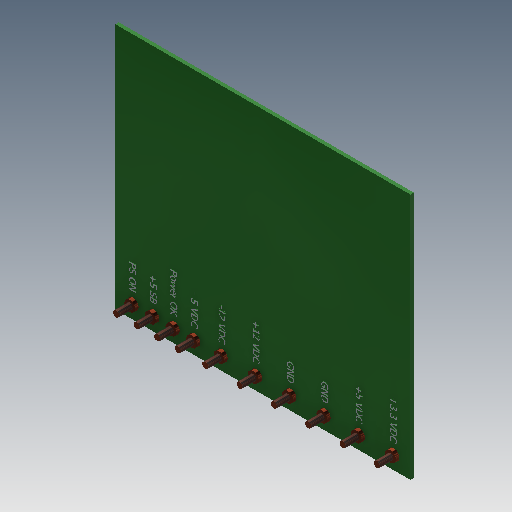
# Autodesk Inventor part: Power Supply PCB
Saved by Autodesk Inventor 2019.1 (Build 231200000, 200)
## iProperties
Created: 2006-09-22
Part Number: Power Supply PCB
Document SubType Name: Modeling
Designer: floress
Density: 1 g/cm^3
Material: Generic
Mass: 25.5294 g
Surface Area: 329.972 cm^2
Volume: 25.5294 cm^3
Appearance: Smooth - Dark Forest Green
Author: floress
Autodesk Inventor part; units mm, degrees
(part 1 of 2)
ref_plane "YZ Plane" through (0, 0, 0) normal (1, 0, 0) x (0, 1, 0)
ref_plane "XZ Plane" through (0, 0, 0) normal (0, 1, 0) x (-1, 0, 0)
ref_plane "XY Plane" through (0, 0, 0) normal (0, 0, 1) x (1, 0, 0)
sketch "Sketch1" plane through (0, 0, 0) normal (0, 0, 1) x (1, 0, 0)
  line L0 (-70.6268, 69.974) -> (65.8982, 69.974)
  line L1 (65.8982, 69.974) -> (65.8982, -44.326)
  line L2 (65.8982, -44.326) -> (-70.6268, -44.326)
  line L3 (-70.6268, -44.326) -> (-70.6268, 69.974)
  circle A0 centre (58.2782, -37.976) radius 2.54
  circle A1 centre (42.4032, -37.976) radius 2.54
  circle A2 centre (26.5282, -37.976) radius 2.54
  circle A3 centre (10.6532, -37.976) radius 2.54
  circle A4 centre (-5.2218, -37.976) radius 2.54
  circle A5 centre (-21.0968, -37.976) radius 2.54
  circle A6 centre (-33.7968, -37.976) radius 2.54
  circle A7 centre (-43.3218, -37.976) radius 2.54
  circle A8 centre (-62.3718, -37.976) radius 2.54
  circle A9 centre (-52.8468, -37.976) radius 2.54
  circle A10 centre (-62.3718, -37.976) radius 1.4224
  circle A11 centre (-52.8468, -37.976) radius 1.4224
  circle A12 centre (-43.3218, -37.976) radius 1.4224
  circle A13 centre (-33.7968, -37.976) radius 1.4224
  circle A14 centre (-21.0968, -37.976) radius 1.4224
  circle A15 centre (-5.2218, -37.976) radius 1.4224
  circle A16 centre (10.6532, -37.976) radius 1.4224
  circle A17 centre (26.5282, -37.976) radius 1.4224
  circle A18 centre (42.4032, -37.976) radius 1.4224
  circle A19 centre (58.2782, -37.976) radius 1.4224
  dimension "d0" = 5.08
  dimension "d1" = 6.35
  dimension "d2" = 7.62
  dimension "d3" = 136.525
  dimension "d4" = 114.3
  dimension "d5" = 15.875
  dimension "d6" = 15.875
  dimension "d7" = 15.875
  dimension "d8" = 15.875
  dimension "d9" = 15.875
  dimension "d10" = 12.7
  dimension "d11" = 9.525
  dimension "d12" = 9.525
  dimension "d13" = 9.525
  dimension "d14" = 2.8448
  constraints: 20 centre point, 18 equal radius, 10 coincident, 9 horizontal alignment, 8 end point, 2 parallel, 1 horizontal, 1 perpendicular
  measures "d0" diameter of A9
  measures "d1" distance from line of L2 A4.centre
  measures "d2" distance from line of L1 A0.centre
  measures "d3" distance of L1.end L2.end
  measures "d4" distance of L0.end L1.end
  measures "d5" distance of A1.centre A0.centre
  measures "d6" distance of A2.centre A1.centre
  measures "d7" distance of A3.centre A2.centre
  measures "d8" distance of A4.centre A3.centre
  measures "d9" distance of A5.centre A4.centre
  measures "d10" distance of A6.centre A5.centre
  measures "d11" distance of A7.centre A6.centre
  measures "d12" distance of A9.centre A7.centre
  measures "d13" distance of A8.centre A9.centre
  measures "d14" diameter of A10
extrude "Extrusion1" add sketch "Sketch1" along normal blind 1.5875 contours L0 L1 L2 L3 | A0 | A1 | A2 | A3 | A4 | A5 | A6 | A7 | A8 | A9 | A10 | A11 | A12 | A13 | A14 | A15 | A16 | A17 | A18 | A19
extrude "Extrusion2" add sketch "Sketch1" along normal blind 3.175 contours A0 | A1 | A2 | A3 | A4 | A5 | A6 | A7 | A8 | A9 | A10 | A11 | A12 | A13 | A14 | A15 | A16 | A17 | A18 | A19
extrude "Extrusion3" add sketch "Sketch1" along normal blind 9.525 contours A10 | A11 | A12 | A13 | A14 | A15 | A16 | A17 | A18 | A19
thread "Thread1" size "4-40 UNC" class "2A" standard "ANSI Unified Screw Threads" full length
thread "Thread2" size "4-40 UNC" class "2A" standard "ANSI Unified Screw Threads" full length
thread "Thread3" size "4-40 UNC" class "2A" standard "ANSI Unified Screw Threads" full length
thread "Thread4" size "4-40 UNC" class "2A" standard "ANSI Unified Screw Threads" full length
thread "Thread5" size "4-40 UNC" class "2A" standard "ANSI Unified Screw Threads" full length
thread "Thread6" size "4-40 UNC" class "2A" standard "ANSI Unified Screw Threads" full length
thread "Thread7" size "4-40 UNC" class "2A" standard "ANSI Unified Screw Threads" full length
thread "Thread8" size "4-40 UNC" class "2A" standard "ANSI Unified Screw Threads" full length
thread "Thread9" size "4-40 UNC" class "2A" standard "ANSI Unified Screw Threads" full length
thread "Thread10" size "4-40 UNC" class "2A" standard "ANSI Unified Screw Threads" full length
sketch "Sketch2" plane through (0, 0, 1.5875) normal (0, 0, 1) x (1, 0, 0)
  circle A0 centre (-52.8468, -37.976) radius 2.54 projected
  circle A1 centre (-62.3718, -37.976) radius 2.54 projected
  circle A2 centre (-43.3218, -37.976) radius 2.54 projected
  circle A3 centre (-33.7968, -37.976) radius 2.54 projected
  circle A4 centre (-21.0968, -37.976) radius 2.54 projected
  circle A5 centre (-5.2218, -37.976) radius 2.54 projected
  circle A6 centre (10.6532, -37.976) radius 2.54 projected
  circle A7 centre (26.5282, -37.976) radius 2.54 projected
  circle A8 centre (42.4032, -37.976) radius 2.54 projected
  circle A9 centre (58.2782, -37.976) radius 2.54 projected
  line L0 (65.8982, 69.974) -> (65.8982, -44.326) projected
  line L1 (59.8664, -14.9782) -> (59.8664, -33.0439) construction
  line L2 (59.8664, -33.0439) -> (56.69, -33.0439) construction
  line L3 (56.69, -33.0439) -> (56.69, -14.9782) construction
  line L4 (56.69, -14.9782) -> (59.8664, -14.9782) construction
  line L5 (43.9914, -14.9782) -> (43.9914, -33.0439) construction
  line L6 (43.9914, -33.0439) -> (40.815, -33.0439) construction
  line L7 (40.815, -33.0439) -> (40.815, -14.9782) construction
  line L8 (40.815, -14.9782) -> (43.9914, -14.9782) construction
  line L9 (28.1164, -14.9782) -> (28.1164, -33.0439) construction
  line L10 (28.1164, -33.0439) -> (24.94, -33.0439) construction
  line L11 (24.94, -33.0439) -> (24.94, -14.9782) construction
  line L12 (24.94, -14.9782) -> (28.1164, -14.9782) construction
  line L13 (9.065, -14.9782) -> (12.2414, -14.9782) construction
  line L14 (12.2414, -14.9782) -> (12.2414, -33.0439) construction
  line L15 (12.2414, -33.0439) -> (9.065, -33.0439) construction
  line L16 (9.065, -33.0439) -> (9.065, -14.9782) construction
  line L17 (-6.81, -14.9782) -> (-3.6336, -14.9782) construction
  line L18 (-3.6336, -14.9782) -> (-3.6336, -33.0439) construction
  line L19 (-3.6336, -33.0439) -> (-6.81, -33.0439) construction
  line L20 (-6.81, -33.0439) -> (-6.81, -14.9782) construction
  line L21 (-60.7836, -14.9782) -> (-60.7836, -33.0439) construction
  line L22 (-60.7836, -33.0439) -> (-63.96, -33.0439) construction
  line L23 (-63.96, -33.0439) -> (-63.96, -14.9782) construction
  line L24 (-63.96, -14.9782) -> (-60.7836, -14.9782) construction
  line L25 (-54.435, -14.9782) -> (-51.2586, -14.9782) construction
  line L26 (-51.2586, -14.9782) -> (-51.2586, -33.0439) construction
  line L27 (-51.2586, -33.0439) -> (-54.435, -33.0439) construction
  line L28 (-54.435, -33.0439) -> (-54.435, -14.9782) construction
  line L29 (-44.91, -14.9782) -> (-41.7336, -14.9782) construction
  line L30 (-41.7336, -14.9782) -> (-41.7336, -33.0439) construction
  line L31 (-41.7336, -33.0439) -> (-44.91, -33.0439) construction
  line L32 (-44.91, -33.0439) -> (-44.91, -14.9782) construction
  line L33 (-35.385, -14.9782) -> (-32.2086, -14.9782) construction
  line L34 (-32.2086, -14.9782) -> (-32.2086, -33.0439) construction
  line L35 (-32.2086, -33.0439) -> (-35.385, -33.0439) construction
  line L36 (-35.385, -33.0439) -> (-35.385, -14.9782) construction
  line L37 (-22.685, -14.9782) -> (-19.5086, -14.9782) construction
  line L38 (-19.5086, -14.9782) -> (-19.5086, -33.0439) construction
  line L39 (-19.5086, -33.0439) -> (-22.685, -33.0439) construction
  line L40 (-22.685, -33.0439) -> (-22.685, -14.9782) construction
  line L41 (57.925, -17.7076) -> (57.925, -16.6751)
  line L42 (57.925, -16.6751) -> (56.8925, -16.6751)
  line L43 (56.8925, -16.6751) -> (56.8925, -16.3342)
  line L44 (56.8925, -16.3342) -> (57.925, -16.3342)
  line L45 (57.925, -16.3342) -> (57.925, -15.3018)
  line L46 (57.925, -15.3018) -> (58.2535, -15.3018)
  line L47 (58.2535, -15.3018) -> (58.2535, -16.3342)
  line L48 (58.2535, -16.3342) -> (59.286, -16.3342)
  line L49 (59.286, -16.3342) -> (59.286, -16.6751)
  line L50 (59.286, -16.6751) -> (58.2535, -16.6751)
  line L51 (58.2535, -16.6751) -> (58.2535, -17.7076)
  line L52 (58.2535, -17.7076) -> (57.925, -17.7076)
  spline S0 degree 2 poles (59.5132, -19.0735) (59.5132, -18.9623) (59.4589, -18.7425) (59.4169, -18.6363) knots 0 0 0 1 2 2 2
  spline S1 degree 2 poles (59.4169, -18.6363) (59.3749, -18.5375) (59.286, -18.3918) (59.2464, -18.335) knots 0 0 0 1 2 2 2
  line L53 (59.2464, -18.335) -> (59.2464, -18.3103)
  line L54 (59.2464, -18.3103) -> (59.6787, -18.3103)
  spline S2 degree 2 poles (59.6787, -18.3103) (59.7503, -18.4436) (59.8664, -18.9006) (59.8664, -19.1056) knots 0 0 0 1 2 2 2
  spline S3 degree 2 poles (59.8664, -19.1056) (59.8664, -19.3131) (59.7824, -19.6218) (59.6935, -19.7478) knots 0 0 0 1 2 2 2
  spline S4 degree 2 poles (59.6935, -19.7478) (59.5972, -19.8812) (59.3181, -20.0195) (59.1304, -20.0195) knots 0 0 0 1 2 2 2
  spline S5 degree 2 poles (59.1304, -20.0195) (58.8784, -20.0195) (58.498, -19.6885) (58.4486, -19.4563) knots 0 0 0 1 2 2 2
  line L55 (58.4486, -19.4563) -> (58.419, -19.4563)
  spline S6 degree 2 poles (58.419, -19.4563) (58.3992, -19.5527) (58.3103, -19.7725) (58.2214, -19.8664) knots 0 0 0 1 2 2 2
  spline S7 degree 2 poles (58.2214, -19.8664) (58.1349, -19.9602) (57.8583, -20.0788) (57.6582, -20.0788) knots 0 0 0 1 2 2 2
  spline S8 degree 2 poles (57.6582, -20.0788) (57.4532, -20.0788) (57.1049, -19.938) (56.9716, -19.8096) knots 0 0 0 1 2 2 2
  spline S9 degree 2 poles (56.9716, -19.8096) (56.8332, -19.6762) (56.69, -19.2983) (56.69, -19.0587) knots 0 0 0 1 2 2 2
  spline S10 degree 2 poles (56.69, -19.0587) (56.69, -18.829) (56.8011, -18.3794) (56.8777, -18.2263) knots 0 0 0 1 2 2 2
  line L56 (56.8777, -18.2263) -> (57.31, -18.2263)
  line L57 (57.31, -18.2263) -> (57.31, -18.2559)
  spline S11 degree 2 poles (57.31, -18.2559) (57.2161, -18.3844) (57.0432, -18.8191) (57.0432, -19.034) knots 0 0 0 1 2 2 2
  spline S12 degree 2 poles (57.0432, -19.034) (57.0432, -19.1599) (57.1222, -19.4119) (57.2136, -19.4959) knots 0 0 0 1 2 2 2
  spline S13 degree 2 poles (57.2136, -19.4959) (57.305, -19.5774) (57.5224, -19.6638) (57.6879, -19.6638) knots 0 0 0 1 2 2 2
  spline S14 degree 2 poles (57.6879, -19.6638) (57.8534, -19.6638) (58.0682, -19.5675) (58.13, -19.481) knots 0 0 0 1 2 2 2
  spline S15 degree 2 poles (58.13, -19.481) (58.1917, -19.3946) (58.2387, -19.1599) (58.2387, -19.0216) knots 0 0 0 1 2 2 2
  line L58 (58.2387, -19.0216) -> (58.2387, -18.8487)
  line L59 (58.2387, -18.8487) -> (58.5771, -18.8487)
  line L60 (58.5771, -18.8487) -> (58.5771, -18.9846)
  spline S16 degree 2 poles (58.5771, -18.9846) (58.5771, -19.2587) (58.8389, -19.6045) (59.0884, -19.6045) knots 0 0 0 1 2 2 2
  spline S17 degree 2 poles (59.0884, -19.6045) (59.2045, -19.6045) (59.3699, -19.5156) (59.4193, -19.444) knots 0 0 0 1 2 2 2
  spline S18 degree 2 poles (59.4193, -19.444) (59.4712, -19.3674) (59.5132, -19.1797) (59.5132, -19.0735) knots 0 0 0 1 2 2 2
  line L61 (56.7542, -21.1928) -> (56.7542, -20.7037)
  line L62 (56.7542, -20.7037) -> (57.3371, -20.7037)
  line L63 (57.3371, -20.7037) -> (57.3371, -21.1928)
  line L64 (57.3371, -21.1928) -> (56.7542, -21.1928)
  spline S19 degree 2 poles (59.5132, -22.6303) (59.5132, -22.5192) (59.4589, -22.2993) (59.4169, -22.1931) knots 0 0 0 1 2 2 2
  spline S20 degree 2 poles (59.4169, -22.1931) (59.3749, -22.0943) (59.286, -21.9486) (59.2464, -21.8918) knots 0 0 0 1 2 2 2
  line L65 (59.2464, -21.8918) -> (59.2464, -21.8671)
  line L66 (59.2464, -21.8671) -> (59.6787, -21.8671)
  spline S21 degree 2 poles (59.6787, -21.8671) (59.7503, -22.0005) (59.8664, -22.4574) (59.8664, -22.6624) knots 0 0 0 1 2 2 2
  spline S22 degree 2 poles (59.8664, -22.6624) (59.8664, -22.8699) (59.7824, -23.1787) (59.6935, -23.3046) knots 0 0 0 1 2 2 2
  spline S23 degree 2 poles (59.6935, -23.3046) (59.5972, -23.438) (59.3181, -23.5763) (59.1304, -23.5763) knots 0 0 0 1 2 2 2
  spline S24 degree 2 poles (59.1304, -23.5763) (58.8784, -23.5763) (58.498, -23.2453) (58.4486, -23.0132) knots 0 0 0 1 2 2 2
  line L67 (58.4486, -23.0132) -> (58.419, -23.0132)
  spline S25 degree 2 poles (58.419, -23.0132) (58.3992, -23.1095) (58.3103, -23.3293) (58.2214, -23.4232) knots 0 0 0 1 2 2 2
  spline S26 degree 2 poles (58.2214, -23.4232) (58.1349, -23.5171) (57.8583, -23.6356) (57.6582, -23.6356) knots 0 0 0 1 2 2 2
  spline S27 degree 2 poles (57.6582, -23.6356) (57.4532, -23.6356) (57.1049, -23.4948) (56.9716, -23.3664) knots 0 0 0 1 2 2 2
  spline S28 degree 2 poles (56.9716, -23.3664) (56.8332, -23.233) (56.69, -22.8551) (56.69, -22.6155) knots 0 0 0 1 2 2 2
  spline S29 degree 2 poles (56.69, -22.6155) (56.69, -22.3858) (56.8011, -21.9362) (56.8777, -21.7831) knots 0 0 0 1 2 2 2
  line L68 (56.8777, -21.7831) -> (57.31, -21.7831)
  line L69 (57.31, -21.7831) -> (57.31, -21.8127)
  spline S30 degree 2 poles (57.31, -21.8127) (57.2161, -21.9412) (57.0432, -22.3759) (57.0432, -22.5908) knots 0 0 0 1 2 2 2
  spline S31 degree 2 poles (57.0432, -22.5908) (57.0432, -22.7168) (57.1222, -22.9687) (57.2136, -23.0527) knots 0 0 0 1 2 2 2
  spline S32 degree 2 poles (57.2136, -23.0527) (57.305, -23.1342) (57.5224, -23.2206) (57.6879, -23.2206) knots 0 0 0 1 2 2 2
  spline S33 degree 2 poles (57.6879, -23.2206) (57.8534, -23.2206) (58.0682, -23.1243) (58.13, -23.0379) knots 0 0 0 1 2 2 2
  spline S34 degree 2 poles (58.13, -23.0379) (58.1917, -22.9514) (58.2387, -22.7168) (58.2387, -22.5784) knots 0 0 0 1 2 2 2
  line L70 (58.2387, -22.5784) -> (58.2387, -22.4055)
  line L71 (58.2387, -22.4055) -> (58.5771, -22.4055)
  line L72 (58.5771, -22.4055) -> (58.5771, -22.5414)
  spline S35 degree 2 poles (58.5771, -22.5414) (58.5771, -22.8156) (58.8389, -23.1614) (59.0884, -23.1614) knots 0 0 0 1 2 2 2
  spline S36 degree 2 poles (59.0884, -23.1614) (59.2045, -23.1614) (59.3699, -23.0724) (59.4193, -23.0008) knots 0 0 0 1 2 2 2
  spline S37 degree 2 poles (59.4193, -23.0008) (59.4712, -22.9242) (59.5132, -22.7365) (59.5132, -22.6303) knots 0 0 0 1 2 2 2
  line L73 (59.8022, -27.7013) -> (56.7542, -26.6515)
  line L74 (56.7542, -26.6515) -> (56.7542, -26.2143)
  line L75 (56.7542, -26.2143) -> (59.8022, -25.1646)
  line L76 (59.8022, -25.1646) -> (59.8022, -25.5993)
  line L77 (59.8022, -25.5993) -> (57.2704, -26.444)
  line L78 (57.2704, -26.444) -> (59.8022, -27.2888)
  line L79 (59.8022, -27.2888) -> (59.8022, -27.7013)
  spline S38 degree 2 poles (58.2757, -30.396) (57.8583, -30.396) (57.1865, -30.0577) (56.9987, -29.7736) knots 0 0 0 1 2 2 2
  spline S39 degree 2 poles (56.9987, -29.7736) (56.853, -29.5414) (56.7542, -29.0647) (56.7542, -28.6942) knots 0 0 0 1 2 2 2
  line L80 (56.7542, -28.6942) -> (56.7542, -27.9927)
  line L81 (56.7542, -27.9927) -> (59.8022, -27.9927)
  line L82 (59.8022, -27.9927) -> (59.8022, -28.6868)
  spline S40 degree 2 poles (59.8022, -28.6868) (59.8022, -29.1166) (59.6738, -29.6056) (59.5601, -29.7785) knots 0 0 0 1 2 2 2
  spline S41 degree 2 poles (59.5601, -29.7785) (59.365, -30.0725) (58.7203, -30.396) (58.2757, -30.396) knots 0 0 0 1 2 2 2
  spline S42 degree 2 poles (58.2807, -29.9737) (58.6314, -29.9737) (59.1279, -29.7415) (59.2687, -29.5118) knots 0 0 0 1 2 2 2
  spline S43 degree 2 poles (59.2687, -29.5118) (59.365, -29.3488) (59.4515, -28.9807) (59.4515, -28.7066) knots 0 0 0 1 2 2 2
  line L83 (59.4515, -28.7066) -> (59.4515, -28.3978)
  line L84 (59.4515, -28.3978) -> (57.1049, -28.3978)
  line L85 (57.1049, -28.3978) -> (57.1049, -28.7066)
  spline S44 degree 2 poles (57.1049, -28.7066) (57.1049, -28.9758) (57.1914, -29.3833) (57.3075, -29.5488) knots 0 0 0 1 2 2 2
  spline S45 degree 2 poles (57.3075, -29.5488) (57.4507, -29.7613) (57.925, -29.9737) (58.2807, -29.9737) knots 0 0 0 1 2 2 2
  spline S46 degree 2 poles (56.6999, -32.0263) (56.6999, -31.7299) (56.8999, -31.2284) (57.1, -31.0457) knots 0 0 0 1 2 2 2
  spline S47 degree 2 poles (57.1, -31.0457) (57.2976, -30.8629) (57.8904, -30.6628) (58.2757, -30.6628) knots 0 0 0 1 2 2 2
  spline S48 degree 2 poles (58.2757, -30.6628) (58.6586, -30.6628) (59.2267, -30.8579) (59.4366, -31.0432) knots 0 0 0 1 2 2 2
  spline S49 degree 2 poles (59.4366, -31.0432) (59.6416, -31.226) (59.8565, -31.7249) (59.8565, -32.0337) knots 0 0 0 1 2 2 2
  spline S50 degree 2 poles (59.8565, -32.0337) (59.8565, -32.1868) (59.8121, -32.456) (59.7775, -32.5697) knots 0 0 0 1 2 2 2
  spline S51 degree 2 poles (59.7775, -32.5697) (59.7454, -32.6685) (59.654, -32.8735) (59.5997, -32.9747) knots 0 0 0 1 2 2 2
  line L86 (59.5997, -32.9747) -> (59.1106, -32.9747)
  line L87 (59.1106, -32.9747) -> (59.1106, -32.9426)
  spline S52 degree 2 poles (59.1106, -32.9426) (59.16, -32.8883) (59.2983, -32.7203) (59.365, -32.5993) knots 0 0 0 1 2 2 2
  spline S53 degree 2 poles (59.365, -32.5993) (59.4292, -32.4832) (59.5107, -32.209) (59.5107, -32.0312) knots 0 0 0 1 2 2 2
  spline S54 degree 2 poles (59.5107, -32.0312) (59.5107, -31.8361) (59.3502, -31.4878) (59.197, -31.3569) knots 0 0 0 1 2 2 2
  spline S55 degree 2 poles (59.197, -31.3569) (59.0414, -31.2284) (58.5697, -31.0852) (58.2757, -31.0852) knots 0 0 0 1 2 2 2
  spline S56 degree 2 poles (58.2757, -31.0852) (57.962, -31.0852) (57.51, -31.2359) (57.3544, -31.3668) knots 0 0 0 1 2 2 2
  spline S57 degree 2 poles (57.3544, -31.3668) (57.2037, -31.4952) (57.0506, -31.8385) (57.0506, -32.0312) knots 0 0 0 1 2 2 2
  spline S58 degree 2 poles (57.0506, -32.0312) (57.0506, -32.2066) (57.1371, -32.5054) (57.2013, -32.6215) knots 0 0 0 1 2 2 2
  spline S59 degree 2 poles (57.2013, -32.6215) (57.2655, -32.7327) (57.3989, -32.8982) (57.4458, -32.9451) knots 0 0 0 1 2 2 2
  line L88 (57.4458, -32.9451) -> (57.4458, -32.9747)
  line L89 (57.4458, -32.9747) -> (56.9617, -32.9747)
  spline S60 degree 2 poles (56.9617, -32.9747) (56.9147, -32.8735) (56.8283, -32.6956) (56.7888, -32.5697) knots 0 0 0 1 2 2 2
  spline S61 degree 2 poles (56.7888, -32.5697) (56.7443, -32.4363) (56.6999, -32.209) (56.6999, -32.0263) knots 0 0 0 1 2 2 2
  line L90 (42.0599, -21.2644) -> (42.0599, -20.2319)
  line L91 (42.0599, -20.2319) -> (41.0274, -20.2319)
  line L92 (41.0274, -20.2319) -> (41.0274, -19.8911)
  line L93 (41.0274, -19.8911) -> (42.0599, -19.8911)
  line L94 (42.0599, -19.8911) -> (42.0599, -18.8586)
  line L95 (42.0599, -18.8586) -> (42.3884, -18.8586)
  line L96 (42.3884, -18.8586) -> (42.3884, -19.8911)
  line L97 (42.3884, -19.8911) -> (43.4208, -19.8911)
  line L98 (43.4208, -19.8911) -> (43.4208, -20.2319)
  line L99 (43.4208, -20.2319) -> (42.3884, -20.2319)
  line L100 (42.3884, -20.2319) -> (42.3884, -21.2644)
  line L101 (42.3884, -21.2644) -> (42.0599, -21.2644)
  spline S62 degree 2 poles (41.8573, -23.6554) (41.6375, -23.6554) (41.2621, -23.5146) (41.1237, -23.3861) knots 0 0 0 1 2 2 2
  spline S63 degree 2 poles (41.1237, -23.3861) (40.9854, -23.2577) (40.8249, -22.8748) (40.8249, -22.6377) knots 0 0 0 1 2 2 2
  spline S64 degree 2 poles (40.8249, -22.6377) (40.8249, -22.4204) (40.9212, -21.9955) (40.9978, -21.8399) knots 0 0 0 1 2 2 2
  line L102 (40.9978, -21.8399) -> (41.43, -21.8399)
  line L103 (41.43, -21.8399) -> (41.43, -21.8695)
  spline S65 degree 2 poles (41.43, -21.8695) (41.3954, -21.9165) (41.3065, -22.0919) (41.267, -22.1981) knots 0 0 0 1 2 2 2
  spline S66 degree 2 poles (41.267, -22.1981) (41.225, -22.3191) (41.1781, -22.5192) (41.1781, -22.6451) knots 0 0 0 1 2 2 2
  spline S67 degree 2 poles (41.1781, -22.6451) (41.1781, -22.7686) (41.267, -23.0008) (41.3633, -23.0848) knots 0 0 0 1 2 2 2
  spline S68 degree 2 poles (41.3633, -23.0848) (41.4547, -23.1614) (41.6968, -23.2404) (41.8598, -23.2404) knots 0 0 0 1 2 2 2
  spline S69 degree 2 poles (41.8598, -23.2404) (42.0228, -23.2404) (42.2303, -23.1515) (42.2995, -23.0675) knots 0 0 0 1 2 2 2
  spline S70 degree 2 poles (42.2995, -23.0675) (42.376, -22.9811) (42.4402, -22.7242) (42.4402, -22.5686) knots 0 0 0 1 2 2 2
  spline S71 degree 2 poles (42.4402, -22.5686) (42.4402, -22.4006) (42.3884, -22.0672) (42.3661, -21.9659) knots 0 0 0 1 2 2 2
  line L104 (42.3661, -21.9659) -> (43.9371, -21.9659)
  line L105 (43.9371, -21.9659) -> (43.9371, -23.6381)
  line L106 (43.9371, -23.6381) -> (43.5789, -23.6381)
  line L107 (43.5789, -23.6381) -> (43.5789, -22.3586)
  line L108 (43.5789, -22.3586) -> (42.7663, -22.3586)
  spline S72 degree 2 poles (42.7663, -22.3586) (42.7762, -22.4327) (42.7836, -22.576) (42.7836, -22.6353) knots 0 0 0 1 2 2 2
  spline S73 degree 2 poles (42.7836, -22.6353) (42.7836, -22.8699) (42.707, -23.1935) (42.5934, -23.3417) knots 0 0 0 1 2 2 2
  spline S74 degree 2 poles (42.5934, -23.3417) (42.4798, -23.4924) (42.134, -23.6554) (41.8573, -23.6554) knots 0 0 0 1 2 2 2
  line L109 (43.9371, -27.7013) -> (40.8891, -26.6515)
  line L110 (40.8891, -26.6515) -> (40.8891, -26.2143)
  line L111 (40.8891, -26.2143) -> (43.9371, -25.1646)
  line L112 (43.9371, -25.1646) -> (43.9371, -25.5993)
  line L113 (43.9371, -25.5993) -> (41.4053, -26.444)
  line L114 (41.4053, -26.444) -> (43.9371, -27.2888)
  line L115 (43.9371, -27.2888) -> (43.9371, -27.7013)
  spline S75 degree 2 poles (42.4106, -30.396) (41.9932, -30.396) (41.3213, -30.0577) (41.1336, -29.7736) knots 0 0 0 1 2 2 2
  spline S76 degree 2 poles (41.1336, -29.7736) (40.9879, -29.5414) (40.8891, -29.0647) (40.8891, -28.6942) knots 0 0 0 1 2 2 2
  line L116 (40.8891, -28.6942) -> (40.8891, -27.9927)
  line L117 (40.8891, -27.9927) -> (43.9371, -27.9927)
  line L118 (43.9371, -27.9927) -> (43.9371, -28.6868)
  spline S77 degree 2 poles (43.9371, -28.6868) (43.9371, -29.1166) (43.8086, -29.6056) (43.695, -29.7785) knots 0 0 0 1 2 2 2
  spline S78 degree 2 poles (43.695, -29.7785) (43.4999, -30.0725) (42.8552, -30.396) (42.4106, -30.396) knots 0 0 0 1 2 2 2
  spline S79 degree 2 poles (42.4155, -29.9737) (42.7663, -29.9737) (43.2628, -29.7415) (43.4036, -29.5118) knots 0 0 0 1 2 2 2
  spline S80 degree 2 poles (43.4036, -29.5118) (43.4999, -29.3488) (43.5863, -28.9807) (43.5863, -28.7066) knots 0 0 0 1 2 2 2
  line L119 (43.5863, -28.7066) -> (43.5863, -28.3978)
  line L120 (43.5863, -28.3978) -> (41.2398, -28.3978)
  line L121 (41.2398, -28.3978) -> (41.2398, -28.7066)
  spline S81 degree 2 poles (41.2398, -28.7066) (41.2398, -28.9758) (41.3263, -29.3833) (41.4424, -29.5488) knots 0 0 0 1 2 2 2
  spline S82 degree 2 poles (41.4424, -29.5488) (41.5856, -29.7613) (42.0599, -29.9737) (42.4155, -29.9737) knots 0 0 0 1 2 2 2
  spline S83 degree 2 poles (40.8347, -32.0263) (40.8347, -31.7299) (41.0348, -31.2284) (41.2349, -31.0457) knots 0 0 0 1 2 2 2
  spline S84 degree 2 poles (41.2349, -31.0457) (41.4325, -30.8629) (42.0253, -30.6628) (42.4106, -30.6628) knots 0 0 0 1 2 2 2
  spline S85 degree 2 poles (42.4106, -30.6628) (42.7935, -30.6628) (43.3616, -30.8579) (43.5715, -31.0432) knots 0 0 0 1 2 2 2
  spline S86 degree 2 poles (43.5715, -31.0432) (43.7765, -31.226) (43.9914, -31.7249) (43.9914, -32.0337) knots 0 0 0 1 2 2 2
  spline S87 degree 2 poles (43.9914, -32.0337) (43.9914, -32.1868) (43.947, -32.456) (43.9124, -32.5697) knots 0 0 0 1 2 2 2
  spline S88 degree 2 poles (43.9124, -32.5697) (43.8803, -32.6685) (43.7889, -32.8735) (43.7345, -32.9747) knots 0 0 0 1 2 2 2
  line L122 (43.7345, -32.9747) -> (43.2455, -32.9747)
  line L123 (43.2455, -32.9747) -> (43.2455, -32.9426)
  spline S89 degree 2 poles (43.2455, -32.9426) (43.2949, -32.8883) (43.4332, -32.7203) (43.4999, -32.5993) knots 0 0 0 1 2 2 2
  spline S90 degree 2 poles (43.4999, -32.5993) (43.5641, -32.4832) (43.6456, -32.209) (43.6456, -32.0312) knots 0 0 0 1 2 2 2
  spline S91 degree 2 poles (43.6456, -32.0312) (43.6456, -31.8361) (43.4851, -31.4878) (43.3319, -31.3569) knots 0 0 0 1 2 2 2
  spline S92 degree 2 poles (43.3319, -31.3569) (43.1763, -31.2284) (42.7045, -31.0852) (42.4106, -31.0852) knots 0 0 0 1 2 2 2
  spline S93 degree 2 poles (42.4106, -31.0852) (42.0969, -31.0852) (41.6449, -31.2359) (41.4893, -31.3668) knots 0 0 0 1 2 2 2
  spline S94 degree 2 poles (41.4893, -31.3668) (41.3386, -31.4952) (41.1855, -31.8385) (41.1855, -32.0312) knots 0 0 0 1 2 2 2
  spline S95 degree 2 poles (41.1855, -32.0312) (41.1855, -32.2066) (41.2719, -32.5054) (41.3362, -32.6215) knots 0 0 0 1 2 2 2
  spline S96 degree 2 poles (41.3362, -32.6215) (41.4004, -32.7327) (41.5338, -32.8982) (41.5807, -32.9451) knots 0 0 0 1 2 2 2
  line L124 (41.5807, -32.9451) -> (41.5807, -32.9747)
  line L125 (41.5807, -32.9747) -> (41.0966, -32.9747)
  spline S97 degree 2 poles (41.0966, -32.9747) (41.0496, -32.8735) (40.9632, -32.6956) (40.9237, -32.5697) knots 0 0 0 1 2 2 2
  spline S98 degree 2 poles (40.9237, -32.5697) (40.8792, -32.4363) (40.8347, -32.209) (40.8347, -32.0263) knots 0 0 0 1 2 2 2
  spline S99 degree 2 poles (24.9548, -26.1896) (24.9548, -25.866) (25.1524, -25.33) (25.3525, -25.1374) knots 0 0 0 1 2 2 2
  spline S100 degree 2 poles (25.3525, -25.1374) (25.555, -24.9447) (26.1528, -24.7397) (26.5405, -24.7397) knots 0 0 0 1 2 2 2
  spline S101 degree 2 poles (26.5405, -24.7397) (26.9086, -24.7397) (27.4915, -24.9472) (27.699, -25.1399) knots 0 0 0 1 2 2 2
  spline S102 degree 2 poles (27.699, -25.1399) (27.8991, -25.3251) (28.1164, -25.8685) (28.1164, -26.1921) knots 0 0 0 1 2 2 2
  spline S103 degree 2 poles (28.1164, -26.1921) (28.1164, -26.3477) (28.072, -26.6293) (28.0324, -26.7577) knots 0 0 0 1 2 2 2
  spline S104 degree 2 poles (28.0324, -26.7577) (28.0028, -26.8615) (27.8941, -27.1134) (27.8546, -27.19) knots 0 0 0 1 2 2 2
  line L126 (27.8546, -27.19) -> (27.3655, -27.19)
  line L127 (27.3655, -27.19) -> (27.3655, -27.1554)
  spline S105 degree 2 poles (27.3655, -27.1554) (27.4322, -27.0788) (27.5533, -26.9183) (27.6224, -26.7701) knots 0 0 0 1 2 2 2
  spline S106 degree 2 poles (27.6224, -26.7701) (27.6842, -26.6466) (27.7657, -26.3279) (27.7657, -26.1451) knots 0 0 0 1 2 2 2
  spline S107 degree 2 poles (27.7657, -26.1451) (27.7657, -25.7055) (27.1037, -25.1621) (26.5529, -25.1621) knots 0 0 0 1 2 2 2
  spline S108 degree 2 poles (26.5529, -25.1621) (26.2466, -25.1621) (25.7872, -25.3053) (25.6291, -25.4412) knots 0 0 0 1 2 2 2
  spline S109 degree 2 poles (25.6291, -25.4412) (25.471, -25.5721) (25.3055, -25.9426) (25.3055, -26.1748) knots 0 0 0 1 2 2 2
  spline S110 degree 2 poles (25.3055, -26.1748) (25.3055, -26.3452) (25.3549, -26.6861) (25.4043, -26.8022) knots 0 0 0 1 2 2 2
  line L128 (25.4043, -26.8022) -> (26.1923, -26.8022)
  line L129 (26.1923, -26.8022) -> (26.1923, -26.0957)
  line L130 (26.1923, -26.0957) -> (26.548, -26.0957)
  line L131 (26.548, -26.0957) -> (26.548, -27.2023)
  line L132 (26.548, -27.2023) -> (25.2166, -27.2023)
  spline S111 degree 2 poles (25.2166, -27.2023) (25.182, -27.1257) (25.0758, -26.8639) (25.0437, -26.7528) knots 0 0 0 1 2 2 2
  spline S112 degree 2 poles (25.0437, -26.7528) (24.9993, -26.6021) (24.9548, -26.36) (24.9548, -26.1896) knots 0 0 0 1 2 2 2
  line L133 (25.0141, -29.8922) -> (25.0141, -29.4377)
  line L134 (25.0141, -29.4377) -> (27.6422, -28.0891)
  line L135 (27.6422, -28.0891) -> (25.0141, -28.0891)
  line L136 (25.0141, -28.0891) -> (25.0141, -27.7111)
  line L137 (25.0141, -27.7111) -> (28.0621, -27.7111)
  line L138 (28.0621, -27.7111) -> (28.0621, -28.2867)
  line L139 (28.0621, -28.2867) -> (25.6489, -29.5143)
  line L140 (25.6489, -29.5143) -> (28.0621, -29.5143)
  line L141 (28.0621, -29.5143) -> (28.0621, -29.8922)
  line L142 (28.0621, -29.8922) -> (25.0141, -29.8922)
  spline S113 degree 2 poles (26.5356, -32.913) (26.1182, -32.913) (25.4463, -32.5746) (25.2586, -32.2905) knots 0 0 0 1 2 2 2
  spline S114 degree 2 poles (25.2586, -32.2905) (25.1129, -32.0584) (25.0141, -31.5817) (25.0141, -31.2112) knots 0 0 0 1 2 2 2
  line L143 (25.0141, -31.2112) -> (25.0141, -30.5097)
  line L144 (25.0141, -30.5097) -> (28.0621, -30.5097)
  line L145 (28.0621, -30.5097) -> (28.0621, -31.2037)
  spline S115 degree 2 poles (28.0621, -31.2037) (28.0621, -31.6335) (27.9336, -32.1226) (27.82, -32.2955) knots 0 0 0 1 2 2 2
  spline S116 degree 2 poles (27.82, -32.2955) (27.6249, -32.5894) (26.9802, -32.913) (26.5356, -32.913) knots 0 0 0 1 2 2 2
  spline S117 degree 2 poles (26.5405, -32.4906) (26.8913, -32.4906) (27.3878, -32.2584) (27.5286, -32.0287) knots 0 0 0 1 2 2 2
  spline S118 degree 2 poles (27.5286, -32.0287) (27.6249, -31.8657) (27.7113, -31.4977) (27.7113, -31.2235) knots 0 0 0 1 2 2 2
  line L146 (27.7113, -31.2235) -> (27.7113, -30.9147)
  line L147 (27.7113, -30.9147) -> (25.3648, -30.9147)
  line L148 (25.3648, -30.9147) -> (25.3648, -31.2235)
  spline S119 degree 2 poles (25.3648, -31.2235) (25.3648, -31.4927) (25.4513, -31.9003) (25.5674, -32.0658) knots 0 0 0 1 2 2 2
  spline S120 degree 2 poles (25.5674, -32.0658) (25.7106, -32.2782) (26.1849, -32.4906) (26.5405, -32.4906) knots 0 0 0 1 2 2 2
  spline S121 degree 2 poles (9.0798, -26.1896) (9.0798, -25.866) (9.2774, -25.33) (9.4775, -25.1374) knots 0 0 0 1 2 2 2
  spline S122 degree 2 poles (9.4775, -25.1374) (9.68, -24.9447) (10.2778, -24.7397) (10.6655, -24.7397) knots 0 0 0 1 2 2 2
  spline S123 degree 2 poles (10.6655, -24.7397) (11.0336, -24.7397) (11.6165, -24.9472) (11.824, -25.1399) knots 0 0 0 1 2 2 2
  spline S124 degree 2 poles (11.824, -25.1399) (12.0241, -25.3251) (12.2414, -25.8685) (12.2414, -26.1921) knots 0 0 0 1 2 2 2
  spline S125 degree 2 poles (12.2414, -26.1921) (12.2414, -26.3477) (12.197, -26.6293) (12.1574, -26.7577) knots 0 0 0 1 2 2 2
  spline S126 degree 2 poles (12.1574, -26.7577) (12.1278, -26.8615) (12.0191, -27.1134) (11.9796, -27.19) knots 0 0 0 1 2 2 2
  line L149 (11.9796, -27.19) -> (11.4905, -27.19)
  line L150 (11.4905, -27.19) -> (11.4905, -27.1554)
  spline S127 degree 2 poles (11.4905, -27.1554) (11.5572, -27.0788) (11.6783, -26.9183) (11.7474, -26.7701) knots 0 0 0 1 2 2 2
  spline S128 degree 2 poles (11.7474, -26.7701) (11.8092, -26.6466) (11.8907, -26.3279) (11.8907, -26.1451) knots 0 0 0 1 2 2 2
  spline S129 degree 2 poles (11.8907, -26.1451) (11.8907, -25.7055) (11.2287, -25.1621) (10.6779, -25.1621) knots 0 0 0 1 2 2 2
  spline S130 degree 2 poles (10.6779, -25.1621) (10.3716, -25.1621) (9.9122, -25.3053) (9.7541, -25.4412) knots 0 0 0 1 2 2 2
  spline S131 degree 2 poles (9.7541, -25.4412) (9.596, -25.5721) (9.4305, -25.9426) (9.4305, -26.1748) knots 0 0 0 1 2 2 2
  spline S132 degree 2 poles (9.4305, -26.1748) (9.4305, -26.3452) (9.4799, -26.6861) (9.5293, -26.8022) knots 0 0 0 1 2 2 2
  line L151 (9.5293, -26.8022) -> (10.3173, -26.8022)
  line L152 (10.3173, -26.8022) -> (10.3173, -26.0957)
  line L153 (10.3173, -26.0957) -> (10.673, -26.0957)
  line L154 (10.673, -26.0957) -> (10.673, -27.2023)
  line L155 (10.673, -27.2023) -> (9.3416, -27.2023)
  spline S133 degree 2 poles (9.3416, -27.2023) (9.307, -27.1257) (9.2008, -26.8639) (9.1687, -26.7528) knots 0 0 0 1 2 2 2
  spline S134 degree 2 poles (9.1687, -26.7528) (9.1243, -26.6021) (9.0798, -26.36) (9.0798, -26.1896) knots 0 0 0 1 2 2 2
  line L156 (9.1391, -29.8922) -> (9.1391, -29.4377)
  line L157 (9.1391, -29.4377) -> (11.7672, -28.0891)
  line L158 (11.7672, -28.0891) -> (9.1391, -28.0891)
  line L159 (9.1391, -28.0891) -> (9.1391, -27.7111)
  line L160 (9.1391, -27.7111) -> (12.1871, -27.7111)
  line L161 (12.1871, -27.7111) -> (12.1871, -28.2867)
  line L162 (12.1871, -28.2867) -> (9.7739, -29.5143)
  line L163 (9.7739, -29.5143) -> (12.1871, -29.5143)
  line L164 (12.1871, -29.5143) -> (12.1871, -29.8922)
  line L165 (12.1871, -29.8922) -> (9.1391, -29.8922)
  spline S135 degree 2 poles (10.6606, -32.913) (10.2432, -32.913) (9.5713, -32.5746) (9.3836, -32.2905) knots 0 0 0 1 2 2 2
  spline S136 degree 2 poles (9.3836, -32.2905) (9.2379, -32.0584) (9.1391, -31.5817) (9.1391, -31.2112) knots 0 0 0 1 2 2 2
  line L166 (9.1391, -31.2112) -> (9.1391, -30.5097)
  line L167 (9.1391, -30.5097) -> (12.1871, -30.5097)
  line L168 (12.1871, -30.5097) -> (12.1871, -31.2037)
  spline S137 degree 2 poles (12.1871, -31.2037) (12.1871, -31.6335) (12.0586, -32.1226) (11.945, -32.2955) knots 0 0 0 1 2 2 2
  spline S138 degree 2 poles (11.945, -32.2955) (11.7499, -32.5894) (11.1052, -32.913) (10.6606, -32.913) knots 0 0 0 1 2 2 2
  spline S139 degree 2 poles (10.6655, -32.4906) (11.0163, -32.4906) (11.5128, -32.2584) (11.6536, -32.0287) knots 0 0 0 1 2 2 2
  spline S140 degree 2 poles (11.6536, -32.0287) (11.7499, -31.8657) (11.8363, -31.4977) (11.8363, -31.2235) knots 0 0 0 1 2 2 2
  line L169 (11.8363, -31.2235) -> (11.8363, -30.9147)
  line L170 (11.8363, -30.9147) -> (9.4898, -30.9147)
  line L171 (9.4898, -30.9147) -> (9.4898, -31.2235)
  spline S141 degree 2 poles (9.4898, -31.2235) (9.4898, -31.4927) (9.5763, -31.9003) (9.6924, -32.0658) knots 0 0 0 1 2 2 2
  spline S142 degree 2 poles (9.6924, -32.0658) (9.8356, -32.2782) (10.3099, -32.4906) (10.6655, -32.4906) knots 0 0 0 1 2 2 2
  line L172 (-5.575, -18.9772) -> (-5.575, -17.9447)
  line L173 (-5.575, -17.9447) -> (-6.6075, -17.9447)
  line L174 (-6.6075, -17.9447) -> (-6.6075, -17.6038)
  line L175 (-6.6075, -17.6038) -> (-5.575, -17.6038)
  line L176 (-5.575, -17.6038) -> (-5.575, -16.5714)
  line L177 (-5.575, -16.5714) -> (-5.2465, -16.5714)
  line L178 (-5.2465, -16.5714) -> (-5.2465, -17.6038)
  line L179 (-5.2465, -17.6038) -> (-4.214, -17.6038)
  line L180 (-4.214, -17.6038) -> (-4.214, -17.9447)
  line L181 (-4.214, -17.9447) -> (-5.2465, -17.9447)
  line L182 (-5.2465, -17.9447) -> (-5.2465, -18.9772)
  line L183 (-5.2465, -18.9772) -> (-5.575, -18.9772)
  line L184 (-6.7458, -21.2471) -> (-6.7458, -19.7602)
  line L185 (-6.7458, -19.7602) -> (-6.4346, -19.7602)
  line L186 (-6.4346, -19.7602) -> (-6.4346, -20.3134)
  line L187 (-6.4346, -20.3134) -> (-4.3919, -20.3134)
  line L188 (-4.3919, -20.3134) -> (-4.3919, -19.7602)
  line L189 (-4.3919, -19.7602) -> (-4.1128, -19.7602)
  spline S143 degree 2 poles (-4.1128, -19.7602) (-4.1128, -20.0738) (-3.9349, -20.3703) (-3.6879, -20.39) knots 0 0 0 1 2 2 2
  line L190 (-3.6879, -20.39) -> (-3.6879, -20.7062)
  line L191 (-3.6879, -20.7062) -> (-6.4346, -20.7062)
  line L192 (-6.4346, -20.7062) -> (-6.4346, -21.2471)
  line L193 (-6.4346, -21.2471) -> (-6.7458, -21.2471)
  line L194 (-6.7458, -23.6875) -> (-6.7458, -21.8078)
  line L195 (-6.7458, -21.8078) -> (-6.3135, -21.8078)
  spline S144 degree 2 poles (-6.3135, -21.8078) (-6.1234, -22.0103) (-5.7701, -22.371) (-5.58, -22.5439) knots 0 0 0 1 2 2 2
  spline S145 degree 2 poles (-5.58, -22.5439) (-5.1971, -22.8921) (-4.7377, -23.1465) (-4.4931, -23.1465) knots 0 0 0 1 2 2 2
  spline S146 degree 2 poles (-4.4931, -23.1465) (-4.3647, -23.1465) (-4.172, -23.0675) (-4.1103, -22.9959) knots 0 0 0 1 2 2 2
  spline S147 degree 2 poles (-4.1103, -22.9959) (-4.0485, -22.9242) (-3.9868, -22.7365) (-3.9868, -22.6229) knots 0 0 0 1 2 2 2
  spline S148 degree 2 poles (-3.9868, -22.6229) (-3.9868, -22.5142) (-4.0411, -22.2919) (-4.0831, -22.1907) knots 0 0 0 1 2 2 2
  spline S149 degree 2 poles (-4.0831, -22.1907) (-4.1177, -22.1042) (-4.2165, -21.9437) (-4.2511, -21.8943) knots 0 0 0 1 2 2 2
  line L196 (-4.2511, -21.8943) -> (-4.2511, -21.872)
  line L197 (-4.2511, -21.872) -> (-3.8164, -21.872)
  spline S150 degree 2 poles (-3.8164, -21.872) (-3.7546, -21.998) (-3.6336, -22.45) (-3.6336, -22.6525) knots 0 0 0 1 2 2 2
  spline S151 degree 2 poles (-3.6336, -22.6525) (-3.6336, -23.0799) (-4.0856, -23.5615) (-4.4709, -23.5615) knots 0 0 0 1 2 2 2
  spline S152 degree 2 poles (-4.4709, -23.5615) (-4.6512, -23.5615) (-4.9526, -23.4775) (-5.081, -23.4034) knots 0 0 0 1 2 2 2
  spline S153 degree 2 poles (-5.081, -23.4034) (-5.2144, -23.3293) (-5.4762, -23.1144) (-5.6022, -22.9959) knots 0 0 0 1 2 2 2
  spline S154 degree 2 poles (-5.6022, -22.9959) (-5.8121, -22.8032) (-6.2617, -22.3314) (-6.3926, -22.1907) knots 0 0 0 1 2 2 2
  line L198 (-6.3926, -22.1907) -> (-6.3926, -23.6875)
  line L199 (-6.3926, -23.6875) -> (-6.7458, -23.6875)
  line L200 (-3.6978, -27.7013) -> (-6.7458, -26.6515)
  line L201 (-6.7458, -26.6515) -> (-6.7458, -26.2143)
  line L202 (-6.7458, -26.2143) -> (-3.6978, -25.1646)
  line L203 (-3.6978, -25.1646) -> (-3.6978, -25.5993)
  line L204 (-3.6978, -25.5993) -> (-6.2296, -26.444)
  line L205 (-6.2296, -26.444) -> (-3.6978, -27.2888)
  line L206 (-3.6978, -27.2888) -> (-3.6978, -27.7013)
  spline S155 degree 2 poles (-5.2243, -30.396) (-5.6417, -30.396) (-6.3135, -30.0577) (-6.5013, -29.7736) knots 0 0 0 1 2 2 2
  spline S156 degree 2 poles (-6.5013, -29.7736) (-6.647, -29.5414) (-6.7458, -29.0647) (-6.7458, -28.6942) knots 0 0 0 1 2 2 2
  line L207 (-6.7458, -28.6942) -> (-6.7458, -27.9927)
  line L208 (-6.7458, -27.9927) -> (-3.6978, -27.9927)
  line L209 (-3.6978, -27.9927) -> (-3.6978, -28.6868)
  spline S157 degree 2 poles (-3.6978, -28.6868) (-3.6978, -29.1166) (-3.8262, -29.6056) (-3.9399, -29.7785) knots 0 0 0 1 2 2 2
  spline S158 degree 2 poles (-3.9399, -29.7785) (-4.135, -30.0725) (-4.7797, -30.396) (-5.2243, -30.396) knots 0 0 0 1 2 2 2
  spline S159 degree 2 poles (-5.2193, -29.9737) (-4.8686, -29.9737) (-4.3721, -29.7415) (-4.2313, -29.5118) knots 0 0 0 1 2 2 2
  spline S160 degree 2 poles (-4.2313, -29.5118) (-4.135, -29.3488) (-4.0485, -28.9807) (-4.0485, -28.7066) knots 0 0 0 1 2 2 2
  line L210 (-4.0485, -28.7066) -> (-4.0485, -28.3978)
  line L211 (-4.0485, -28.3978) -> (-6.3951, -28.3978)
  line L212 (-6.3951, -28.3978) -> (-6.3951, -28.7066)
  spline S161 degree 2 poles (-6.3951, -28.7066) (-6.3951, -28.9758) (-6.3086, -29.3833) (-6.1925, -29.5488) knots 0 0 0 1 2 2 2
  spline S162 degree 2 poles (-6.1925, -29.5488) (-6.0493, -29.7613) (-5.575, -29.9737) (-5.2193, -29.9737) knots 0 0 0 1 2 2 2
  spline S163 degree 2 poles (-6.8001, -32.0263) (-6.8001, -31.7299) (-6.6001, -31.2284) (-6.4, -31.0457) knots 0 0 0 1 2 2 2
  spline S164 degree 2 poles (-6.4, -31.0457) (-6.2024, -30.8629) (-5.6096, -30.6628) (-5.2243, -30.6628) knots 0 0 0 1 2 2 2
  spline S165 degree 2 poles (-5.2243, -30.6628) (-4.8414, -30.6628) (-4.2733, -30.8579) (-4.0634, -31.0432) knots 0 0 0 1 2 2 2
  spline S166 degree 2 poles (-4.0634, -31.0432) (-3.8584, -31.226) (-3.6435, -31.7249) (-3.6435, -32.0337) knots 0 0 0 1 2 2 2
  spline S167 degree 2 poles (-3.6435, -32.0337) (-3.6435, -32.1868) (-3.6879, -32.456) (-3.7225, -32.5697) knots 0 0 0 1 2 2 2
  spline S168 degree 2 poles (-3.7225, -32.5697) (-3.7546, -32.6685) (-3.846, -32.8735) (-3.9003, -32.9747) knots 0 0 0 1 2 2 2
  line L213 (-3.9003, -32.9747) -> (-4.3894, -32.9747)
  line L214 (-4.3894, -32.9747) -> (-4.3894, -32.9426)
  spline S169 degree 2 poles (-4.3894, -32.9426) (-4.34, -32.8883) (-4.2017, -32.7203) (-4.135, -32.5993) knots 0 0 0 1 2 2 2
  spline S170 degree 2 poles (-4.135, -32.5993) (-4.0708, -32.4832) (-3.9893, -32.209) (-3.9893, -32.0312) knots 0 0 0 1 2 2 2
  spline S171 degree 2 poles (-3.9893, -32.0312) (-3.9893, -31.8361) (-4.1498, -31.4878) (-4.303, -31.3569) knots 0 0 0 1 2 2 2
  spline S172 degree 2 poles (-4.303, -31.3569) (-4.4586, -31.2284) (-4.9303, -31.0852) (-5.2243, -31.0852) knots 0 0 0 1 2 2 2
  spline S173 degree 2 poles (-5.2243, -31.0852) (-5.538, -31.0852) (-5.99, -31.2359) (-6.1456, -31.3668) knots 0 0 0 1 2 2 2
  spline S174 degree 2 poles (-6.1456, -31.3668) (-6.2963, -31.4952) (-6.4494, -31.8385) (-6.4494, -32.0312) knots 0 0 0 1 2 2 2
  spline S175 degree 2 poles (-6.4494, -32.0312) (-6.4494, -32.2066) (-6.3629, -32.5054) (-6.2987, -32.6215) knots 0 0 0 1 2 2 2
  spline S176 degree 2 poles (-6.2987, -32.6215) (-6.2345, -32.7327) (-6.1011, -32.8982) (-6.0542, -32.9451) knots 0 0 0 1 2 2 2
  line L215 (-6.0542, -32.9451) -> (-6.0542, -32.9747)
  line L216 (-6.0542, -32.9747) -> (-6.5383, -32.9747)
  spline S177 degree 2 poles (-6.5383, -32.9747) (-6.5853, -32.8735) (-6.6717, -32.6956) (-6.7112, -32.5697) knots 0 0 0 1 2 2 2
  spline S178 degree 2 poles (-6.7112, -32.5697) (-6.7557, -32.4363) (-6.8001, -32.209) (-6.8001, -32.0263) knots 0 0 0 1 2 2 2
  line L217 (-21.4722, -19.1155) -> (-21.4722, -17.962)
  line L218 (-21.4722, -17.962) -> (-21.1017, -17.962)
  line L219 (-21.1017, -17.962) -> (-21.1017, -19.1155)
  line L220 (-21.1017, -19.1155) -> (-21.4722, -19.1155)
  line L221 (-22.6208, -21.2471) -> (-22.6208, -19.7602)
  line L222 (-22.6208, -19.7602) -> (-22.3096, -19.7602)
  line L223 (-22.3096, -19.7602) -> (-22.3096, -20.3134)
  line L224 (-22.3096, -20.3134) -> (-20.2669, -20.3134)
  line L225 (-20.2669, -20.3134) -> (-20.2669, -19.7602)
  line L226 (-20.2669, -19.7602) -> (-19.9878, -19.7602)
  spline S179 degree 2 poles (-19.9878, -19.7602) (-19.9878, -20.0738) (-19.8099, -20.3703) (-19.5629, -20.39) knots 0 0 0 1 2 2 2
  line L227 (-19.5629, -20.39) -> (-19.5629, -20.7062)
  line L228 (-19.5629, -20.7062) -> (-22.3096, -20.7062)
  line L229 (-22.3096, -20.7062) -> (-22.3096, -21.2471)
  line L230 (-22.3096, -21.2471) -> (-22.6208, -21.2471)
  line L231 (-22.6208, -23.6875) -> (-22.6208, -21.8078)
  line L232 (-22.6208, -21.8078) -> (-22.1885, -21.8078)
  spline S180 degree 2 poles (-22.1885, -21.8078) (-21.9984, -22.0103) (-21.6451, -22.371) (-21.455, -22.5439) knots 0 0 0 1 2 2 2
  spline S181 degree 2 poles (-21.455, -22.5439) (-21.0721, -22.8921) (-20.6127, -23.1465) (-20.3681, -23.1465) knots 0 0 0 1 2 2 2
  spline S182 degree 2 poles (-20.3681, -23.1465) (-20.2397, -23.1465) (-20.047, -23.0675) (-19.9853, -22.9959) knots 0 0 0 1 2 2 2
  spline S183 degree 2 poles (-19.9853, -22.9959) (-19.9235, -22.9242) (-19.8618, -22.7365) (-19.8618, -22.6229) knots 0 0 0 1 2 2 2
  spline S184 degree 2 poles (-19.8618, -22.6229) (-19.8618, -22.5142) (-19.9161, -22.2919) (-19.9581, -22.1907) knots 0 0 0 1 2 2 2
  spline S185 degree 2 poles (-19.9581, -22.1907) (-19.9927, -22.1042) (-20.0915, -21.9437) (-20.1261, -21.8943) knots 0 0 0 1 2 2 2
  line L233 (-20.1261, -21.8943) -> (-20.1261, -21.872)
  line L234 (-20.1261, -21.872) -> (-19.6914, -21.872)
  spline S186 degree 2 poles (-19.6914, -21.872) (-19.6296, -21.998) (-19.5086, -22.45) (-19.5086, -22.6525) knots 0 0 0 1 2 2 2
  spline S187 degree 2 poles (-19.5086, -22.6525) (-19.5086, -23.0799) (-19.9606, -23.5615) (-20.3459, -23.5615) knots 0 0 0 1 2 2 2
  spline S188 degree 2 poles (-20.3459, -23.5615) (-20.5262, -23.5615) (-20.8276, -23.4775) (-20.956, -23.4034) knots 0 0 0 1 2 2 2
  spline S189 degree 2 poles (-20.956, -23.4034) (-21.0894, -23.3293) (-21.3512, -23.1144) (-21.4772, -22.9959) knots 0 0 0 1 2 2 2
  spline S190 degree 2 poles (-21.4772, -22.9959) (-21.6871, -22.8032) (-22.1367, -22.3314) (-22.2676, -22.1907) knots 0 0 0 1 2 2 2
  line L235 (-22.2676, -22.1907) -> (-22.2676, -23.6875)
  line L236 (-22.2676, -23.6875) -> (-22.6208, -23.6875)
  line L237 (-19.5728, -27.7013) -> (-22.6208, -26.6515)
  line L238 (-22.6208, -26.6515) -> (-22.6208, -26.2143)
  line L239 (-22.6208, -26.2143) -> (-19.5728, -25.1646)
  line L240 (-19.5728, -25.1646) -> (-19.5728, -25.5993)
  line L241 (-19.5728, -25.5993) -> (-22.1046, -26.444)
  line L242 (-22.1046, -26.444) -> (-19.5728, -27.2888)
  line L243 (-19.5728, -27.2888) -> (-19.5728, -27.7013)
  spline S191 degree 2 poles (-21.0993, -30.396) (-21.5167, -30.396) (-22.1885, -30.0577) (-22.3763, -29.7736) knots 0 0 0 1 2 2 2
  spline S192 degree 2 poles (-22.3763, -29.7736) (-22.522, -29.5414) (-22.6208, -29.0647) (-22.6208, -28.6942) knots 0 0 0 1 2 2 2
  line L244 (-22.6208, -28.6942) -> (-22.6208, -27.9927)
  line L245 (-22.6208, -27.9927) -> (-19.5728, -27.9927)
  line L246 (-19.5728, -27.9927) -> (-19.5728, -28.6868)
  spline S193 degree 2 poles (-19.5728, -28.6868) (-19.5728, -29.1166) (-19.7012, -29.6056) (-19.8149, -29.7785) knots 0 0 0 1 2 2 2
  spline S194 degree 2 poles (-19.8149, -29.7785) (-20.01, -30.0725) (-20.6547, -30.396) (-21.0993, -30.396) knots 0 0 0 1 2 2 2
  spline S195 degree 2 poles (-21.0943, -29.9737) (-20.7436, -29.9737) (-20.2471, -29.7415) (-20.1063, -29.5118) knots 0 0 0 1 2 2 2
  spline S196 degree 2 poles (-20.1063, -29.5118) (-20.01, -29.3488) (-19.9235, -28.9807) (-19.9235, -28.7066) knots 0 0 0 1 2 2 2
  line L247 (-19.9235, -28.7066) -> (-19.9235, -28.3978)
  line L248 (-19.9235, -28.3978) -> (-22.2701, -28.3978)
  line L249 (-22.2701, -28.3978) -> (-22.2701, -28.7066)
  spline S197 degree 2 poles (-22.2701, -28.7066) (-22.2701, -28.9758) (-22.1836, -29.3833) (-22.0675, -29.5488) knots 0 0 0 1 2 2 2
  spline S198 degree 2 poles (-22.0675, -29.5488) (-21.9243, -29.7613) (-21.45, -29.9737) (-21.0943, -29.9737) knots 0 0 0 1 2 2 2
  spline S199 degree 2 poles (-22.6751, -32.0263) (-22.6751, -31.7299) (-22.4751, -31.2284) (-22.275, -31.0457) knots 0 0 0 1 2 2 2
  spline S200 degree 2 poles (-22.275, -31.0457) (-22.0774, -30.8629) (-21.4846, -30.6628) (-21.0993, -30.6628) knots 0 0 0 1 2 2 2
  spline S201 degree 2 poles (-21.0993, -30.6628) (-20.7164, -30.6628) (-20.1483, -30.8579) (-19.9384, -31.0432) knots 0 0 0 1 2 2 2
  spline S202 degree 2 poles (-19.9384, -31.0432) (-19.7334, -31.226) (-19.5185, -31.7249) (-19.5185, -32.0337) knots 0 0 0 1 2 2 2
  spline S203 degree 2 poles (-19.5185, -32.0337) (-19.5185, -32.1868) (-19.5629, -32.456) (-19.5975, -32.5697) knots 0 0 0 1 2 2 2
  spline S204 degree 2 poles (-19.5975, -32.5697) (-19.6296, -32.6685) (-19.721, -32.8735) (-19.7753, -32.9747) knots 0 0 0 1 2 2 2
  line L250 (-19.7753, -32.9747) -> (-20.2644, -32.9747)
  line L251 (-20.2644, -32.9747) -> (-20.2644, -32.9426)
  spline S205 degree 2 poles (-20.2644, -32.9426) (-20.215, -32.8883) (-20.0767, -32.7203) (-20.01, -32.5993) knots 0 0 0 1 2 2 2
  spline S206 degree 2 poles (-20.01, -32.5993) (-19.9458, -32.4832) (-19.8643, -32.209) (-19.8643, -32.0312) knots 0 0 0 1 2 2 2
  spline S207 degree 2 poles (-19.8643, -32.0312) (-19.8643, -31.8361) (-20.0248, -31.4878) (-20.178, -31.3569) knots 0 0 0 1 2 2 2
  spline S208 degree 2 poles (-20.178, -31.3569) (-20.3336, -31.2284) (-20.8053, -31.0852) (-21.0993, -31.0852) knots 0 0 0 1 2 2 2
  spline S209 degree 2 poles (-21.0993, -31.0852) (-21.413, -31.0852) (-21.865, -31.2359) (-22.0206, -31.3668) knots 0 0 0 1 2 2 2
  spline S210 degree 2 poles (-22.0206, -31.3668) (-22.1713, -31.4952) (-22.3244, -31.8385) (-22.3244, -32.0312) knots 0 0 0 1 2 2 2
  spline S211 degree 2 poles (-22.3244, -32.0312) (-22.3244, -32.2066) (-22.2379, -32.5054) (-22.1737, -32.6215) knots 0 0 0 1 2 2 2
  spline S212 degree 2 poles (-22.1737, -32.6215) (-22.1095, -32.7327) (-21.9761, -32.8982) (-21.9292, -32.9451) knots 0 0 0 1 2 2 2
  line L252 (-21.9292, -32.9451) -> (-21.9292, -32.9747)
  line L253 (-21.9292, -32.9747) -> (-22.4133, -32.9747)
  spline S213 degree 2 poles (-22.4133, -32.9747) (-22.4603, -32.8735) (-22.5467, -32.6956) (-22.5862, -32.5697) knots 0 0 0 1 2 2 2
  spline S214 degree 2 poles (-22.5862, -32.5697) (-22.6307, -32.4363) (-22.6751, -32.209) (-22.6751, -32.0263) knots 0 0 0 1 2 2 2
  line L254 (-34.1624, -20.0936) -> (-34.1624, -18.9401)
  line L255 (-34.1624, -18.9401) -> (-33.7919, -18.9401)
  line L256 (-33.7919, -18.9401) -> (-33.7919, -20.0936)
  line L257 (-33.7919, -20.0936) -> (-34.1624, -20.0936)
  spline S215 degree 2 poles (-34.3427, -23.6554) (-34.5625, -23.6554) (-34.9379, -23.5146) (-35.0763, -23.3861) knots 0 0 0 1 2 2 2
  spline S216 degree 2 poles (-35.0763, -23.3861) (-35.2146, -23.2577) (-35.3751, -22.8748) (-35.3751, -22.6377) knots 0 0 0 1 2 2 2
  spline S217 degree 2 poles (-35.3751, -22.6377) (-35.3751, -22.4204) (-35.2788, -21.9955) (-35.2022, -21.8399) knots 0 0 0 1 2 2 2
  line L258 (-35.2022, -21.8399) -> (-34.77, -21.8399)
  line L259 (-34.77, -21.8399) -> (-34.77, -21.8695)
  spline S218 degree 2 poles (-34.77, -21.8695) (-34.8046, -21.9165) (-34.8935, -22.0919) (-34.933, -22.1981) knots 0 0 0 1 2 2 2
  spline S219 degree 2 poles (-34.933, -22.1981) (-34.975, -22.3191) (-35.0219, -22.5192) (-35.0219, -22.6451) knots 0 0 0 1 2 2 2
  spline S220 degree 2 poles (-35.0219, -22.6451) (-35.0219, -22.7686) (-34.933, -23.0008) (-34.8367, -23.0848) knots 0 0 0 1 2 2 2
  spline S221 degree 2 poles (-34.8367, -23.0848) (-34.7453, -23.1614) (-34.5032, -23.2404) (-34.3402, -23.2404) knots 0 0 0 1 2 2 2
  spline S222 degree 2 poles (-34.3402, -23.2404) (-34.1772, -23.2404) (-33.9697, -23.1515) (-33.9005, -23.0675) knots 0 0 0 1 2 2 2
  spline S223 degree 2 poles (-33.9005, -23.0675) (-33.824, -22.9811) (-33.7598, -22.7242) (-33.7598, -22.5686) knots 0 0 0 1 2 2 2
  spline S224 degree 2 poles (-33.7598, -22.5686) (-33.7598, -22.4006) (-33.8116, -22.0672) (-33.8339, -21.9659) knots 0 0 0 1 2 2 2
  line L260 (-33.8339, -21.9659) -> (-32.2629, -21.9659)
  line L261 (-32.2629, -21.9659) -> (-32.2629, -23.6381)
  line L262 (-32.2629, -23.6381) -> (-32.6211, -23.6381)
  line L263 (-32.6211, -23.6381) -> (-32.6211, -22.3586)
  line L264 (-32.6211, -22.3586) -> (-33.4337, -22.3586)
  spline S225 degree 2 poles (-33.4337, -22.3586) (-33.4238, -22.4327) (-33.4164, -22.576) (-33.4164, -22.6353) knots 0 0 0 1 2 2 2
  spline S226 degree 2 poles (-33.4164, -22.6353) (-33.4164, -22.8699) (-33.493, -23.1935) (-33.6066, -23.3417) knots 0 0 0 1 2 2 2
  spline S227 degree 2 poles (-33.6066, -23.3417) (-33.7202, -23.4924) (-34.066, -23.6554) (-34.3427, -23.6554) knots 0 0 0 1 2 2 2
  line L265 (-32.2629, -27.7013) -> (-35.3109, -26.6515)
  line L266 (-35.3109, -26.6515) -> (-35.3109, -26.2143)
  line L267 (-35.3109, -26.2143) -> (-32.2629, -25.1646)
  line L268 (-32.2629, -25.1646) -> (-32.2629, -25.5993)
  line L269 (-32.2629, -25.5993) -> (-34.7947, -26.444)
  line L270 (-34.7947, -26.444) -> (-32.2629, -27.2888)
  line L271 (-32.2629, -27.2888) -> (-32.2629, -27.7013)
  spline S228 degree 2 poles (-33.7894, -30.396) (-34.2068, -30.396) (-34.8787, -30.0577) (-35.0664, -29.7736) knots 0 0 0 1 2 2 2